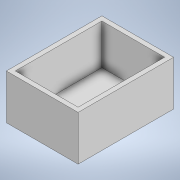
# Autodesk Inventor part: ProkladkaA
Saved by Autodesk Inventor 2022 (Build 260153000, 153)
## iProperties
Created: 2023-08-16
Part Number: ProkladkaA
Material: Generic
Document SubType Name: Modeling
Designer: Kippi
Density: 1 g/cm^3
Appearance: Default
Author: Kippi
Autodesk Inventor part; units mm, degrees
ref_plane "YZ Plane" through (0, 0, 0) normal (1, 0, 0) x (0, 1, 0)
ref_plane "XZ Plane" through (0, 0, 0) normal (0, 1, 0) x (-1, 0, 0)
ref_plane "XY Plane" through (0, 0, 0) normal (0, 0, 1) x (1, 0, 0)
sketch "Sketch1" plane through (0, 0, 0) normal (0, 1, 0) x (-1, 0, 0)
  line L0 (56.8, 106.5) -> (-103.2, 106.5)
  line L1 (-103.2, 106.5) -> (-103.2, -106.5)
  line L2 (-103.2, -106.5) -> (56.8, -106.5)
  line L3 (56.8, -106.5) -> (56.8, 106.5)
  point P0 (0, 0)
  dimension "d0" = 213
  dimension "d1" = 160
  constraints: 8 end point, 2 parallel, 1 horizontal, 1 perpendicular
  measures "d0" distance of L2.end L0.start
  measures "d1" distance of L0.start L0.end
extrude "Extrusion1" add sketch "Sketch1" along normal blind 100
shell "Shell1" thickness 10 removed faces 1 at (49.8667, 100, 35.5)
body "Solid1"
